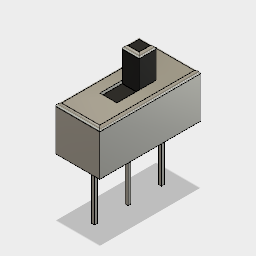
Vertical slide switch SS-12D00G3 High Knob 3mm SPDT v2 (Autodesk Fusion 360 design; units mm, degrees)
Autodesk Fusion 360 part; units mm, degrees
sketch "Sketch1" plane through (0, 0, 0) normal (0, 1, 0) x (1, 0, 0)
  line L0 (1.885, 4.295) -> (-1.885, 4.295)
  line L1 (-1.885, 4.295) -> (-1.885, -4.295)
  line L2 (-1.885, -4.295) -> (1.885, -4.295)
  line L3 (1.885, -4.295) -> (1.885, 4.295)
  line L4 (1.885, 4.295) -> (-1.885, -4.295) construction
  line L5 (-1.885, 4.295) -> (1.885, -4.295) construction
  dimension "d1" = 3.77
  dimension "d2" = 8.59
  measures "d1" distance of L1.end L2.end
  measures "d2" distance of L0.end L1.end
extrude "Extrude1" add sketch "Sketch1" along normal blind 3.77
sketch "Sketch2" plane through (0, 3.77, 0) normal (0, 1, 0) x (-1, 0, 0)
  line L0 (-1.885, 4.295) -> (-1.885, -4.295)
  line L1 (-1.885, -4.295) -> (1.885, -4.295)
  line L2 (1.885, -4.295) -> (1.885, 4.295)
  line L3 (1.885, 4.295) -> (-1.885, 4.295)
  line L4 (0.725, 1.675) -> (-0.725, 1.675)
  line L5 (-0.725, 1.675) -> (-0.725, -1.675)
  line L6 (-0.725, -1.675) -> (0.725, -1.675)
  line L7 (0.725, -1.675) -> (0.725, 1.675)
  line L8 (0.725, 1.675) -> (-0.725, -1.675) construction
  line L9 (-0.725, 1.675) -> (0.725, -1.675) construction
  dimension "d5" = 1.45
  dimension "d6" = 3.35
  measures "d5" distance of L5.end L6.end
  measures "d6" distance of L4.end L5.end
extrude "Extrude2" cut sketch "Sketch2" against normal blind 0.25 contours L4 L5 L6 L7
sketch "Sketch3" plane through (0, 3.52, 0) normal (0, 1, 0) x (-1, 0, 0)
  line L0 (0.725, -1.675) -> (0.725, 1.675)
  line L1 (0.725, 1.675) -> (-0.725, 1.675)
  line L2 (-0.725, 1.675) -> (-0.725, -1.675)
  line L3 (-0.725, -1.675) -> (0.725, -1.675)
  line L4 (0.725, -1.675) -> (-0.725, -1.675)
  line L5 (-0.725, -1.675) -> (-0.725, -0.225)
  line L6 (-0.725, -0.225) -> (0.725, -0.225)
  line L7 (0.725, -0.225) -> (0.725, -1.675)
  dimension "d9" = 1.45
  dimension "d10" = 1.45
  measures "d9" distance of L0.start L2.end
  measures "d10" distance of L0.start L6.end
extrude "Extrude3" add sketch "Sketch3" along normal blind 2.82 contours L0 L2 L3 L4 L5 L6 L7
sketch "Sketch4" plane through (0, 0, 0) normal (0, -1, 0) x (1, 0, 0)
  line L0 (1.885, -4.295) -> (1.885, 4.295)
  line L1 (1.885, 4.295) -> (-1.885, 4.295)
  line L2 (-1.885, 4.295) -> (-1.885, -4.295)
  line L3 (-1.885, -4.295) -> (1.885, -4.295)
  line L4 (0, -4.295) -> (0, 4.295) construction
  line L5 (1.885, 0) -> (-1.885, 0) construction
  line L6 (0.125, -0.125) -> (-0.125, -0.125)
  line L7 (-0.125, -0.125) -> (-0.125, 0.125)
  line L8 (-0.125, 0.125) -> (0.125, 0.125)
  line L9 (0.125, 0.125) -> (0.125, -0.125)
  line L10 (0.125, -0.125) -> (-0.125, 0.125) construction
  line L11 (-0.125, -0.125) -> (0.125, 0.125) construction
  line L12 (0.125, 2.7383) -> (-0.125, 2.7383)
  line L13 (-0.125, 2.7383) -> (-0.125, 2.9883)
  line L14 (-0.125, 2.9883) -> (0.125, 2.9883)
  line L15 (0.125, 2.9883) -> (0.125, 2.7383)
  line L16 (0.125, 2.7383) -> (-0.125, 2.9883) construction
  line L17 (-0.125, 2.7383) -> (0.125, 2.9883) construction
  line L18 (0.125, -2.9883) -> (0.125, -2.7383)
  line L19 (0.125, -2.7383) -> (-0.125, -2.7383)
  line L20 (-0.125, -2.7383) -> (-0.125, -2.9883)
  line L21 (-0.125, -2.9883) -> (0.125, -2.9883)
  point P0 (0, 2.8633)
  point P1 (0, -2.8633)
  dimension "d14" = 0.25
  dimension "d15" = 0.25
  dimension "d16" = 0.25
  dimension "d17" = 0.25
  dimension "d18" = 2.8633
  measures "d14" distance of L7.end L8.end
  measures "d15" distance of L6.end L7.end
  measures "d16" distance of L12.end L13.end
  measures "d17" distance of L13.end L14.end
  measures "d18" distance of origin P0
extrude "Extrude4" add sketch "Sketch4" along normal blind 4.91 contours L6 L7 L8 L9 | L12 L13 L14 L15 | L18 L19 L20 L21
fillet "Fillet1" radius 0.25 4 edges at (1.885, 3.77, 0) (0, 3.77, 4.295) (0, 3.77, -4.295) (-1.885, 3.77, 0)
fillet "Fillet2" radius 0.25 4 edges at (0.725, 6.34, -0.95) (0, 6.34, -1.675) (-0.725, 6.34, -0.95) (0, 6.34, -0.225)
